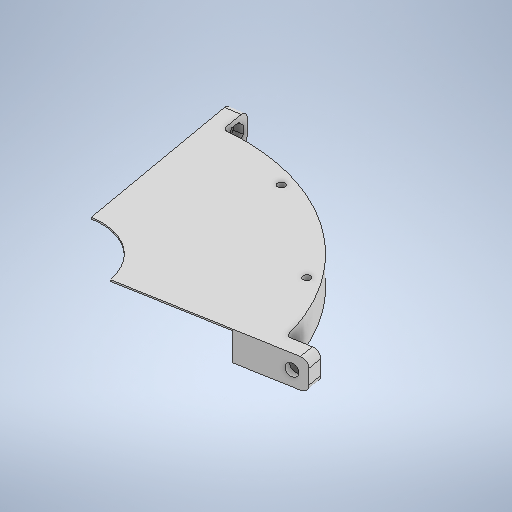
# Autodesk Inventor part: Cylinder Spacer 25mm_Q2+4
Saved by Autodesk Inventor 2025 (Build 290162000, 162)
## iProperties
Created: 2024-04-28
Part Number: Cylinder Spacer 25mm_Q2+4
Material: Generic
Document SubType Name: Modeling
Designer: Thienan Hoang
Density: 1 g/cm^3
Appearance: Default
Author: Thienan Hoang
Autodesk Inventor part; units mm, degrees
ref_plane "YZ Plane" through (0, 0, 0) normal (1, 0, 0) x (0, 1, 0)
ref_plane "XZ Plane" through (0, 0, 0) normal (0, 1, 0) x (-1, 0, 0)
ref_plane "XY Plane" through (0, 0, 0) normal (0, 0, 1) x (1, 0, 0)
sketch "Sketch1" plane through (0, 0, 0) normal (0, 1, 0) x (-1, 0, 0)
  circle A0 centre (0, 0) radius 135
  circle A1 centre (0, 0) radius 110
  dimension "d0" = 270
  dimension "d1" = 220
  constraints: 2 centre point, 2 coincident
  measures "d0" diameter of A0
  measures "d1" diameter of A1
extrude "Extrusion1" add sketch "Sketch1" along normal mid plane 20
sketch "Sketch2" plane through (0, 10, 0) normal (0, 1, 0) x (1, 0, 0)
  circle A0 centre (0, 0) radius 37.5
  circle A1 centre (0, 0) radius 135
  dimension "d4" = 75
  dimension "d20" = 270
  constraints: 2 centre point, 2 coincident
  measures "d4" diameter of A0
  measures "d20" diameter of A1
extrude "Extrusion2" add sketch "Sketch2" against normal blind 1
sketch "Sketch3" plane through (0, 10, 0) normal (0, 1, 0) x (1, 0, 0)
  circle A0 centre (0, 0) radius 127.5
  circle A1 centre (127.5, 0) radius 2.5
  circle A2 centre (103.1497, 74.9426) radius 2.5
  circle A3 centre (39.3997, 121.2597) radius 2.5
  circle A4 centre (-39.3997, 121.2597) radius 2.5
  circle A5 centre (-103.1497, 74.9426) radius 2.5
  circle A6 centre (-127.5, 0) radius 2.5
  circle A7 centre (-103.1497, -74.9426) radius 2.5
  circle A8 centre (-39.3997, -121.2597) radius 2.5
  circle A9 centre (39.3997, -121.2597) radius 2.5
  circle A10 centre (103.1497, -74.9426) radius 2.5
  dimension "d7" = 255
  dimension "d8" = 5
  dimension "d11" = 360
  constraints: 10 centre point, 1 coincident, 1 horizontal alignment, 23 other
  measures "d8" diameter of A1
hole "Hole1" at (127.5, 10, 0) at (103.1497, 10, 74.9426) at (39.3997, 10, 121.2597) at (-39.3997, 10, 121.2597) at (-103.1497, 10, 74.9426) at (-127.5, 10, 0) at (-103.1497, 10, -74.9426) at (-39.3997, 10, -121.2597) at (39.3997, 10, -121.2597) at (103.1497, 10, -74.9426) direction (0, -1, 0) diameter 5 end through all
sketch "Sketch4" plane through (0, -10, 0) normal (0, -1, 0) x (1, 0, 0)
  circle A0 centre (0, 0) radius 135
  line L0 (0, 0) -> (132.949, -23.4425)
  line L1 (0, 0) -> (135, 0) construction
  line L2 (0, 0) -> (-23.4425, -132.949)
  circle A1 centre (0, 0) radius 135 projected
  line L3 (0, 0) -> (135, 0) construction
  line L4 (0, 0) -> (-132.949, 23.4425)
  dimension "d21" = 135
  dimension "d22" = 10
  dimension "d23" = 100
  constraints: 10 end point, 2 equal length, 2 horizontal, 2 point on circle, 1 centre point, 1 coincident, 1 point on line
  measures "d21" distance of L0.start L0.end
  measures "d22" angle of L0 L1
  measures "d23" angle of L2 L3
extrude "Extrusion3" cut sketch "Sketch4" against normal through all contours A0 L0 L4 | L4 L2 A0
sketch "Sketch5" plane through (-23.4425, -10, -132.949) normal (-0.9848, 0, 0.1736) x (0.1736, 0, 0.9848)
  line L0 (135, 20) -> (0, 20) projected
  line L1 (2.5, 20) -> (-15, 20)
  line L2 (-20, 15) -> (-20, 5)
  line L3 (-15, 0) -> (2.5, 0)
  line L4 (2.5, 0) -> (2.5, 20)
  line L5 (0, 0) -> (0, 20) projected
  arc A0 (-20, 5) -> (-15, 0) centre (-15, 5) ccw
  arc A1 (-15, 20) -> (-20, 15) centre (-15, 15) ccw
  point P0 (135, 10)
  point P1 (-20, 0)
  point P2 (-20, 20)
  point P3 (0, 20)
  dimension "d26" = 22.5
  dimension "d27" = 20
  dimension "d28" = 20
  dimension "d29" = 5
  constraints: 8 end point, 5 point on line, 4 point on circle, 4 tangent, 2 centre point, 2 parallel, 1 equal radius, 1 horizontal, 1 perpendicular
  measures "d26" distance of L3.end point (-20, 0)
  measures "d27" distance of point (-20, 0) point (-20, 20)
  measures "d28" distance between parallel lines of L5 L2
  measures "d29" radius of A0
extrude "Extrusion4" add sketch "Sketch5" against normal blind 10
fillet "Fillet1" radius 2.5 1 edges at (-13.53, 0, -134.3203)
sketch "Sketch6" plane through (132.949, -10, -23.4425) normal (0.1736, 0, 0.9848) x (0.9848, 0, -0.1736)
  line L0 (-122.7273, 0) -> (0, 0) projected
  line L1 (-2.5, 0) -> (15, 0)
  line L2 (20, 5) -> (20, 15)
  line L3 (15, 20) -> (-2.5, 20)
  line L4 (-2.5, 20) -> (-2.5, 0)
  line L5 (0, 20) -> (0, 0) projected
  arc A0 (20, 15) -> (15, 20) centre (15, 15) ccw
  arc A1 (15, 0) -> (20, 5) centre (15, 5) ccw
  point P0 (-135, 10)
  point P1 (20, 20)
  point P2 (20, 0)
  point P3 (0, 0)
  dimension "d33" = 22.5
  dimension "d34" = 20
  dimension "d35" = 20
  dimension "d36" = 5
  constraints: 8 end point, 5 point on line, 4 point on circle, 4 tangent, 2 centre point, 2 parallel, 1 equal radius, 1 horizontal, 1 perpendicular
  measures "d33" distance of L3.end point (20, 20)
  measures "d34" distance of point (20, 20) point (20, 0)
  measures "d35" distance between parallel lines of L5 L2
  measures "d36" radius of A0
extrude "Extrusion5" add sketch "Sketch6" against normal blind 10
fillet "Fillet2" radius 2.5 1 edges at (130.8473, 0, -33.2262)
sketch "Sketch7" plane through (-13.5944, -10, -134.6855) normal (0.9848, 0, -0.1736) x (-0.1736, 0, -0.9848)
  line L0 (16.6, 12.7338) -> (16.6, 7.2662)
  line L1 (16.6, 7.2662) -> (12.7338, 3.4)
  line L2 (12.7338, 3.4) -> (7.2662, 3.4)
  line L3 (7.2662, 3.4) -> (3.4, 7.2662)
  line L4 (3.4, 7.2662) -> (3.4, 12.7338)
  line L5 (3.4, 12.7338) -> (7.2662, 16.6)
  line L6 (7.2662, 16.6) -> (12.7338, 16.6)
  line L7 (12.7338, 16.6) -> (16.6, 12.7338)
  line L8 (20, 5) -> (20, 15) projected
  line L9 (1.9306, 0) -> (15, 0) projected
  point P0 (-135, 10)
  point P1 (10, 10)
  point P2 (20, 10)
  dimension "d40" = 10
  dimension "d41" = 10
  dimension "d42" = 13.2
  constraints: 16 end point, 1 midpoint, 1 vertical, 17 other
  measures "d40" distance of point (20, 10) point (10, 10)
  measures "d41" distance from line of L9 point (10, 10)
  measures "d42" distance between parallel lines of L4 L0
extrude "Extrusion6" cut sketch "Sketch7" against normal blind 6
sketch "Sketch8" plane through (-19.5033, -10, -133.6436) normal (0.9848, 0, -0.1736) x (-0.1736, 0, -0.9848)
  line L0 (1.9306, 0) -> (15, 0) projected
  line L1 (20, 5) -> (20, 15) projected
  point P0 (-135, 10)
  point P1 (10, 10)
  dimension "d45" = 10
  dimension "d46" = 10
  measures "d45" distance from line of L0 point (10, 10)
  measures "d46" distance from line of L1 point (10, 10)
hole "Hole2" at (-21.2398, 0, -143.4917) direction (-0.9848, 0, 0.1736) diameter 8.2 end through all
sketch "Sketch9" plane through (131.2126, -10, -33.2906) normal (-0.1736, 0, -0.9848) x (-0.9848, 0, 0.1736)
  line L0 (-20, 15) -> (-20, 5) projected
  line L1 (-1.9306, 20) -> (-15, 20) projected
  point P0 (135, 10)
  point P1 (-10, 10)
  dimension "d54" = 10
  dimension "d55" = 10
  measures "d54" distance from line of L0 point (-10, 10)
  measures "d55" distance from line of L1 point (-10, 10)
hole "Hole3" at (141.0606, 0, -35.0271) direction (0.1736, 0, 0.9848) diameter 8.2 end through all counterbore diameter 13.2 counterbore depth 6
body "Solid1"
